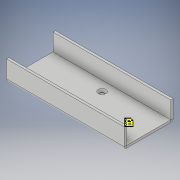
# Autodesk Inventor part: uchannel
Saved by Autodesk Inventor 2017 (Build 210142000, 142)
## iProperties
Created: 2018-03-08
Part Number: uchannel
Material: Generic
Document SubType Name: Sheet Metal
Designer: Zara
Density: 1 g/cm^3
Sheet Metal Rule: Default
Appearance: Default
Author: Zara
Autodesk Inventor part; units mm, degrees
ref_plane "YZ Plane" through (0, 0, 0) normal (1, 0, 0) x (0, 1, 0)
ref_plane "XZ Plane" through (0, 0, 0) normal (0, 1, 0) x (-1, 0, 0)
ref_plane "XY Plane" through (0, 0, 0) normal (0, 0, 1) x (1, 0, 0)
sketch "Sketch2" plane through (0, 0, 0) normal (0, 1, 0) x (-1, 0, 0)
  line L0 (90.4875, -192.0875) -> (-61.9125, -192.0875)
  line L1 (-61.9125, -192.0875) -> (-61.9125, -249.2375)
  line L2 (-61.9125, -249.2375) -> (90.4875, -249.2375)
  line L3 (90.4875, -249.2375) -> (90.4875, -192.0875)
  dimension "d5" = 152.4
  dimension "d6" = 57.15
  measures "d5" distance of L1.end L2.end
  measures "d6" distance of L2.end L0.start
extrude "Plate1" add sketch "Sketch2" along normal blind 3.175
sketch "Sketch3" plane through (61.9125, 3.176, -192.0865) normal (0, 0, 1) x (1, 0, 0)
  line L0 (-152.4, 0) -> (0, 0)
  line L1 (0, 0) -> (0, 22.224)
  line L2 (0, 22.224) -> (-152.4, 22.224)
  line L3 (-152.4, 22.224) -> (-152.4, 0)
  constraints: 6 end point, 1 horizontal, 1 perpendicular, 1 vertical
edge flange "Flange1" height 25.4 angle 90 thickness 3.175 bend radius 0 thickness toward (0, 0, 1) relief tear relief width 3.175 relief depth 1.5875 corner gap 3.175 corner form 0 edges at (-14.2875, 3.175, -192.0875) (-14.2875, 3.175, -249.2375) wall of the first edge with corners at (-90.4875, 3.176, -192.0865) (61.9125, 3.176, -192.0865) (61.9125, 25.4, -192.0865) (-90.4875, 25.4, -192.0865)
bend "Bend1"
corner "Corner1"
sketch "Sketch4" plane through (0, 3.175, 0) normal (0, 1, 0) x (1, 0, 0)
  line L0 (-14.2875, 204.7865) -> (-14.2875, 236.5365) construction
  line L1 (-90.4875, 188.9115) -> (61.9125, 188.9115) construction
  line L2 (-90.4875, 192.0875) -> (-90.4875, 249.2375) construction
  point P0 (0, 0)
  dimension "d20" = 31.75
  dimension "d21" = 15.875
  dimension "d22" = 76.2
  constraints: 2 end point, 1 vertical
  measures "d20" distance of L0.start L0.end
  measures "d21" distance from line of L1 L0.start
  measures "d22" distance between parallel lines of L0 L2
hole "Hole1" at (-14.2875, 3.175, -204.7865) at (-14.2875, 3.175, -236.5365) direction (0, -1, 0) diameter 5.1054 end through all countersink diameter 9.779 countersink angle 82 clearance for "Flat Head Machine Screw (82)" size "#10" standard "Ansi Unified Screw Threads"
equation "\"d10\" = BendReliefWidth"
equation "\"d11\" = BendReliefDepth"
equation "\"d12\" = MinimumRemnant"
equation "\"d13\" = BendRadius"
equation "\"d17\" = CornerReliefSize"
equation "\"d18\" = GapSize"
equation "\"d19\" = JacobiRadiusSize"
equation "\"BendRadius\" = Thickness"
equation "\"BendReliefWidth\" = Thickness"
equation "\"BendReliefDepth\" = 0.5 * Thickness"
equation "\"CornerReliefSize\" = 4 * Thickness"
equation "\"MinimumRemnant\" = 2 * Thickness"
equation "\"TransitionRadius\" = BendRadius"
equation "\"JacobiRadiusSize\" = BendRadius"
equation "\"GapSize\" = Thickness"
equation "\"d9\" = BendRadius"
equation "\"Thickness\" = 3.175"
body "Solid2"
